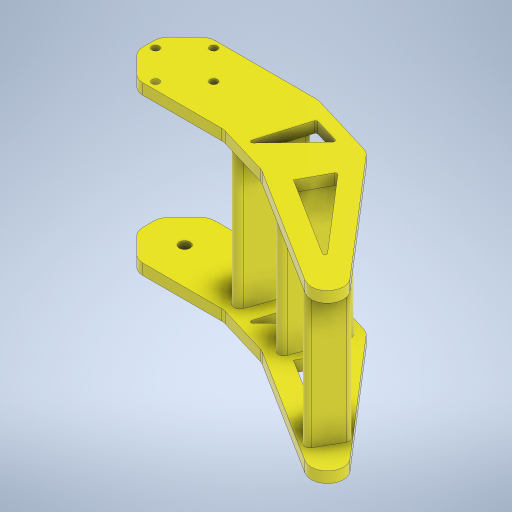
# Autodesk Inventor part: leg_part
Saved by Autodesk Inventor 2024 (Build 280153000, 153)
## iProperties
Created: 2024-02-16
Part Number: leg_part
Material: Generic
Document SubType Name: Modeling
Designer: kamil
Density: 1 g/cm^3
Appearance: Default
Author: kamil
Autodesk Inventor part; units mm, degrees
ref_plane "YZ Plane" through (0, 0, 0) normal (1, 0, 0) x (0, 1, 0)
ref_plane "XZ Plane" through (0, 0, 0) normal (0, 1, 0) x (-1, 0, 0)
ref_plane "XY Plane" through (0, 0, 0) normal (0, 0, 1) x (1, 0, 0)
sketch "Sketch1" plane through (0, 0, 0) normal (0, 1, 0) x (-1, 0, 0)
  line L0 (-11.4129, 10) -> (10.3431, 10)
  line L1 (20, 2) -> (20, -2)
  line L2 (10.3431, -10) -> (-17.4129, -10)
  line L3 (-20, -10) -> (-20, 10)
  line L4 (20, -10) -> (-20, 10) construction
  line L5 (20, 10) -> (-20, -10) construction
  line L6 (13.1716, -8.8284) -> (17.6284, -4.3716)
  line L7 (13.1716, 8.8284) -> (17.6284, 4.3716)
  line L8 (18.8, 1.5431) -> (18.8, -1.5431)
  arc A0 (18.8, 1.5431) -> (17.6284, 4.3716) centre (14.8, 1.5431) ccw
  arc A1 (17.6284, -4.3716) -> (18.8, -1.5431) centre (14.8, -1.5431) ccw
  arc A2 (13.1716, 8.8284) -> (10.3431, 10) centre (10.3431, 6) ccw
  arc A3 (10.3431, -10) -> (13.1716, -8.8284) centre (10.3431, -6) ccw
  line L9 (-18, -10) -> (-12, 10)
  line L10 (-12.5623, 10.1687) -> (-26.3566, 14.307)
  line L11 (-33.8781, 16.5634) -> (-39.8781, -3.4366)
  line L12 (-35.8836, -4.6349) -> (-18.5623, -9.8313)
  line L13 (-26.8781, 14.4634) -> (-37.0046, -4.2986)
  line L14 (-27.3388, 14.7536) -> (-59.1142, 34.7654)
  line L15 (-37.7675, -3.4111) -> (-65.2661, 28.5779)
  arc A4 (-12.5623, 10.1687) -> (-11.4129, 10) centre (-11.4129, 14) ccw
  arc A5 (-18.5623, -9.8313) -> (-17.4129, -10) centre (-17.4129, -6) ccw
  arc A6 (-27.3388, 14.7536) -> (-26.3566, 14.307) centre (-25.2072, 18.1383) ccw
  arc A7 (-37.7675, -3.4111) -> (-35.8836, -4.6349) centre (-34.7342, -0.8036) ccw
  arc A8 (-59.1142, 34.7654) -> (-65.2661, 28.5779) centre (-61.5814, 31.0663) ccw
  line L16 (18.8, 0) -> (8.8, 0)
  circle A9 centre (0.8, 0) radius 1.025
  circle A10 centre (8.8, -8) radius 1.025
  circle A11 centre (16.8, 0) radius 1.025
  circle A12 centre (8.8, 8) radius 1.025
  line L17 (-23.0219, -4.861) -> (-29.7868, -2.8316)
  line L18 (-22.3993, -4.5258) -> (-18.4228, 8.7292)
  line L19 (-19.263, 9.2186) -> (-30.0044, -2.007)
  arc A13 (-23.0219, -4.861) -> (-22.3993, -4.5258) centre (-22.8782, -4.3821) ccw
  arc A14 (-30.0044, -2.007) -> (-29.7868, -2.8316) centre (-29.6432, -2.3526) ccw
  arc A15 (-18.4228, 8.7292) -> (-19.263, 9.2186) centre (-18.9017, 8.8729) ccw
  line L20 (-37.6066, 5.1132) -> (-33.634, 12.4734)
  line L21 (-33.634, 12.4734) -> (-55.2323, 26.0758)
  line L22 (-55.8779, 25.3268) -> (-38.4257, 5.0247)
  arc A16 (-38.4257, 5.0247) -> (-37.6066, 5.1132) centre (-38.0466, 5.3506) ccw
  arc A17 (-55.2323, 26.0758) -> (-55.8779, 25.3268) centre (-55.4988, 25.6528) ccw
  point P0 (0, 0)
  point P1 (0, 0)
  point P2 (12, -10)
  point P3 (12, 10)
  point P4 (20, 10)
  point P5 (18.8, 3.2)
  point P6 (18.8, -3.2)
  point P7 (-37.9518, 4.4734)
  point P8 (-35.6203, 8.7933)
  dimension "d0" = 40
  dimension "d1" = 20
  dimension "d32" = 8
  dimension "d33" = 8
  dimension "d34" = 8
  dimension "d35" = 8
  dimension "d43" = 1.2
  dimension "d46" = 4
  dimension "d47" = 2
  dimension "d48" = 8
  dimension "d49" = 3
  dimension "d50" = 7
  dimension "d51" = 43.3541
  dimension "d52" = 32.617
  dimension "d53" = 4
  dimension "d54" = 10
  dimension "d55" = 2.05
  dimension "d56" = 8
  dimension "d59" = 360
  dimension "d79" = 0.5
  dimension "d80" = 8
  dimension "d81" = 5
  dimension "d82" = 5
  dimension "d83" = 0.5
  constraints: 46 end point, 33 point on line, 28 point on circle, 26 tangent, 18 centre point, 9 equal radius, 6 parallel, 3 midpoint, 2 horizontal, 2 perpendicular, 1 coincident, 1 vertical, 9 other
  measures "d0" distance of L4.start L3.start
  measures "d1" distance of L5.start L4.start
  measures "d32" distance of point (12, -10) point (20, -10)
  measures "d33" distance of L1.end point (20, -10)
  measures "d34" distance of point (12, 10) point (20, 10)
  measures "d35" distance of L1.start point (20, 10)
  measures "d43" distance between parallel lines of L8 L1
  measures "d46" radius of A0
  measures "d47" distance from line of L3 L9.start
  measures "d48" distance of L3.end L9.end
  measures "d49" distance from line of L11 L13.end
  measures "d50" horizontal distance of L11.start L13.start
  measures "d51" distance of L13.end L15.end
  measures "d52" angle of L12 L15
  measures "d53" radius of A4
  measures "d54" distance of L16.start L16.end
  measures "d55" diameter of A9
  measures "d56" distance of A9.centre L16.end
  measures "d79" radius of A13
  measures "d80" vertical distance of point (-37.952, 4.473) L20.end
  measures "d81" distance from line of point (-35.62, 8.793) L13
  measures "d82" distance between parallel lines of L15 L22
  measures "d83" radius of A16
extrude "Extrusion1" add sketch "Sketch1" along normal blind 3
sketch "Sketch8" plane through (0, 0, 0) normal (0, -1, 0) x (1, 0, 0)
  arc A0 (17.4129, -10) -> (18.5623, -9.8313) centre (17.4129, -6) ccw projected
  line L0 (-13.1716, -8.8284) -> (-17.6284, -4.3716) projected
  arc A1 (35.8836, -4.6349) -> (37.7675, -3.4111) centre (34.7342, -0.8036) ccw projected
  circle A2 centre (34.7342, -0.8036) radius 1.5
  circle A3 centre (30.2342, 11.6964) radius 1.5
  line L1 (65.2661, 28.5779) -> (37.7675, -3.4111) projected
  line L2 (27.3388, 14.7536) -> (59.1142, 34.7654) projected
  line L3 (15.9075, -6.542) -> (11.4075, 5.958)
  line L4 (14.4183, 7.042) -> (18.9183, -5.458)
  arc A4 (15.9075, -6.542) -> (18.9183, -5.458) centre (17.4129, -6) ccw
  arc A5 (14.4183, 7.042) -> (11.4075, 5.958) centre (12.9129, 6.5) ccw
  line L5 (34.7342, -0.8036) -> (30.2342, 11.6964) construction
  line L6 (36.1456, -0.2955) -> (31.6456, 12.2045)
  line L7 (28.8229, 11.1883) -> (33.3229, -1.3117)
  arc A6 (33.3229, -1.3117) -> (36.1456, -0.2955) centre (34.7342, -0.8036) ccw
  arc A7 (31.6456, 12.2045) -> (28.8229, 11.1883) centre (30.2342, 11.6964) ccw
  line L8 (59.3782, 24.0575) -> (55.8591, 30.2331) construction
  line L9 (60.5121, 24.7036) -> (56.993, 30.8792)
  line L10 (54.7253, 29.587) -> (58.2444, 23.4114)
  arc A8 (58.2444, 23.4114) -> (60.5121, 24.7036) centre (59.3782, 24.0575) ccw
  arc A9 (56.993, 30.8792) -> (54.7253, 29.587) centre (55.8591, 30.2331) ccw
  point P0 (0, 0)
  point P1 (17.9938, -9.9576)
  point P2 (15.1629, 0.25)
  point P3 (32.4842, 5.4464)
  point P4 (57.6187, 27.1453)
  dimension "d64" = 3
  dimension "d69" = 3
  dimension "d70" = 4.5
  dimension "d71" = 12.5
  dimension "d88" = 1.6
  constraints: 20 end point, 13 point on circle, 12 tangent, 8 centre point, 3 parallel, 2 coincident, 2 midpoint, 1 concentric
  measures "d64" diameter of A2
  measures "d69" diameter of A3
  measures "d70" horizontal distance of L5.end A2.centre
  measures "d71" vertical distance of L5.end A2.centre
  measures "d88" radius of A4
extrude "Extrusion7" add sketch "Sketch8" along normal blind 40
extrude "Extrusion8" add sketch "Sketch1" against normal blind 3 from surface at -40 contours A11 L16 | L16 A11 | L0 A2 L7 A0 L8 A1 L6 A3 L2 A5 L12 A7 L15 A8 L14 A6 L10 A4 | A9 | A10 | A12
sketch "Sketch10" plane through (-10.3431, -43, -10) normal (0, -1, 0) x (1, 0, 0)
  line L0 (-8.4569, 8.4569) -> (-8.4569, 11.5431) projected
  line L1 (-8.4569, 10) -> (1.5431, 10)
  circle A0 centre (1.5431, 10) radius 1.5
  point P0 (10.3431, 10)
  dimension "d84" = 10
  dimension "d85" = 3
  constraints: 2 end point, 1 centre point, 1 coincident, 1 horizontal, 1 midpoint
  measures "d84" distance of L1.start L1.end
  measures "d85" diameter of A0
extrude "Extrusion9" cut sketch "Sketch10" against normal blind 3
equation "\"d33\" = d32"
equation "\"d34\" = d32"
equation "\"d35\" = d34"
body "Solid1"
